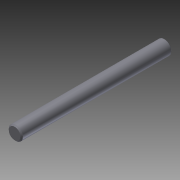
# Autodesk Inventor part: 276-2181-010 Rev1
Saved by Autodesk Inventor 2013 (Build 170138000, 138)
## iProperties
Category: Motors
Company: Autodesk Inc.
Created: 2012-01-28
Part Number: 276-2181-010 Rev1
Material: Steel, Mild
Document SubType Name: Modeling
Designer: Autodesk Inc.
Density: 7.86 g/cm^3
Catalog Web Link: http://www.vexrobotics.com/276-2181.html
Vendor: VEX
Mass: 0.221286 g
Surface Area: 0.781225 cm^2
Volume: 0.0281535 cm^3
Author: Autodesk Inc.
Autodesk Inventor part; units mm, degrees
ref_plane "YZ Plane" through (0, 0, 0) normal (1, 0, 0) x (0, 1, 0)
ref_plane "XZ Plane" through (0, 0, 0) normal (0, 1, 0) x (-1, 0, 0)
ref_plane "XY Plane" through (0, 0, 0) normal (0, 0, 1) x (1, 0, 0)
sketch "Sketch1" plane through (0, 0, 0) normal (0, 0, 1) x (1, 0, 0)
  circle A0 centre (0, 0) radius 0.7493
  dimension "d0" = 1.4986
  constraints: 1 centre point, 1 coincident
  measures "d0" diameter of A0
extrude "Extrusion1" add sketch "Sketch1" against normal blind 16.002
chamfer "Chamfer1" distance 0.127 angle 45 2 edges at (-0.7493, 0, 0) (-0.7493, 0, -16.002)
body "Solid1"
